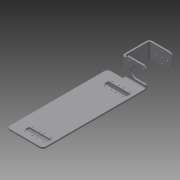
# Autodesk Inventor part: Base
Saved by Autodesk Inventor 2015 (Build 190159000, 159)
## iProperties
Created: 2015-12-09
Part Number: Base
Material: Generic
Document SubType Name: Sheet Metal
Designer: Nick
Density: 1 g/cm^3
Sheet Metal Rule: Default
Appearance: Default
Author: Nick
Autodesk Inventor part; units mm, degrees
ref_plane "YZ Plane" through (0, 0, 0) normal (1, 0, 0) x (0, 1, 0)
ref_plane "XZ Plane" through (0, 0, 0) normal (0, 1, 0) x (-1, 0, 0)
ref_plane "XY Plane" through (0, 0, 0) normal (0, 0, 1) x (1, 0, 0)
sketch "Sketch1" plane through (0, 0, 0) normal (0, 1, 0) x (-1, 0, 0)
  line L0 (0, 0) -> (0, -208.3054)
  line L1 (0, 0) -> (0, 0)
  line L2 (6.35, 6.35) -> (6.35, 6.35)
  line L3 (6.35, 6.35) -> (70.4596, 6.35)
  line L4 (70.4596, 6.35) -> (76.8096, 6.35)
  line L5 (76.8096, 0) -> (76.8096, -201.9554)
  line L6 (76.8096, -208.3054) -> (70.4596, -208.3054)
  line L7 (70.4596, -208.3054) -> (43.6118, -208.3054)
  line L8 (43.6118, -208.3054) -> (43.6118, -217.6526)
  line L9 (43.6118, -217.6526) -> (43.6118, -249.9614)
  line L10 (0, -208.3054) -> (0, -217.6526)
  line L11 (0, -217.6526) -> (43.6118, -217.6526)
  line L12 (0, -208.3054) -> (43.6118, -208.3054)
  line L13 (43.6118, -212.979) -> (0, -212.979)
  arc A0 (70.4596, -208.3054) -> (76.8096, -201.9554) centre (70.4596, -201.9554) ccw
  arc A1 (76.8096, 0) -> (70.4596, 6.35) centre (70.4596, 0) ccw
  arc A2 (6.35, 6.35) -> (0, 0) centre (6.35, 0) ccw
  line L14 (43.6118, -249.9614) -> (43.6118, -253.9492)
  line L15 (0, -253.9492) -> (0, -249.9614)
  line L16 (0, -249.9614) -> (43.6118, -249.9614)
  line L17 (0, -249.9614) -> (0, -217.6526)
  circle A3 centre (20.574, -232.791) radius 12.7
  line L18 (20.574, -245.491) -> (0, -245.491)
  line L19 (20.574, -220.091) -> (0, -220.091)
  line L20 (0, -249.9614) -> (3.9878, -253.9492)
  line L21 (43.6118, -249.9614) -> (39.624, -253.9492)
  line L22 (3.9878, -253.9492) -> (39.624, -253.9492)
  circle A4 centre (5.9436, -248.3104) radius 1.4859
  line L23 (5.9436, -248.3104) -> (36.3728, -248.3104)
  circle A5 centre (36.3728, -248.3104) radius 1.4859
  line L24 (43.6118, -217.6526) -> (52.959, -217.6526)
  line L25 (52.959, -217.6526) -> (52.959, -249.9614)
  line L26 (52.959, -249.9614) -> (43.6118, -249.9614)
  line L27 (48.2854, -249.9614) -> (48.2854, -217.6526)
  line L28 (52.959, -217.6526) -> (96.9518, -217.6526)
  line L29 (96.9518, -217.6526) -> (96.9518, -249.9614)
  line L30 (96.9518, -249.9614) -> (52.959, -249.9614)
  line L31 (96.9518, -249.9614) -> (106.299, -249.9614)
  line L32 (106.299, -249.9614) -> (106.299, -217.6526)
  line L33 (106.299, -217.6526) -> (96.9518, -217.6526)
  line L34 (101.6254, -217.6526) -> (101.6254, -249.9614)
  line L35 (106.299, -217.6526) -> (143.5608, -217.6526)
  line L36 (143.5608, -217.6526) -> (143.5608, -249.9614)
  line L37 (143.5608, -249.9614) -> (106.299, -249.9614)
  line L38 (143.5608, -249.9614) -> (143.5608, -249.9614)
  line L39 (149.9108, -243.6114) -> (149.9108, -224.0026)
  line L40 (143.5608, -217.6526) -> (143.5608, -217.6526)
  arc A6 (149.9108, -224.0026) -> (143.5608, -217.6526) centre (143.5608, -224.0026) ccw
  arc A7 (143.5608, -249.9614) -> (149.9108, -243.6114) centre (143.5608, -243.6114) ccw
  circle A8 centre (128.8542, -233.807) radius 1.9939
  circle A9 centre (117.5512, -233.807) radius 1.4859
  circle A10 centre (128.8542, -245.11) radius 1.4859
  circle A11 centre (140.1572, -233.807) radius 1.4859
  circle A12 centre (128.8542, -222.504) radius 1.4859
  line L41 (0, -208.3054) -> (70.4596, -208.3054)
  arc A13 (70.4596, -208.3054) -> (76.8096, -201.9554) centre (70.4596, -201.9554) ccw
  line L42 (43.6118, -249.9614) -> (39.624, -253.9492)
  line L43 (3.9878, -253.9492) -> (39.624, -253.9492)
  line L44 (0, -249.9614) -> (3.9878, -253.9492)
  line L45 (0, -249.9614) -> (43.6118, -249.9614)
  line L46 (5.9944, -9.398) -> (5.9944, -18.4912)
  line L47 (5.9944, -18.4912) -> (53.8988, -18.4912)
  line L48 (53.8988, -18.4912) -> (53.8988, -9.398)
  line L49 (53.8988, -9.398) -> (5.9944, -9.398)
  line L50 (9.2964, -6.7056) -> (11.8872, -6.7056)
  line L51 (11.8872, -6.7056) -> (11.8872, -5.1562)
  line L52 (11.8872, -5.1562) -> (9.2964, -5.1562)
  line L53 (9.2964, -5.1562) -> (9.2964, -6.7056)
  line L54 (23.9268, -6.7056) -> (26.5176, -6.7056)
  line L55 (26.5176, -6.7056) -> (26.5176, -5.1562)
  line L56 (26.5176, -5.1562) -> (23.9268, -5.1562)
  line L57 (23.9268, -5.1562) -> (23.9268, -6.7056)
  line L58 (29.9466, -9.398) -> (29.9466, -18.4912)
  line L59 (53.8988, -13.9446) -> (41.6179, -13.9446)
  line L60 (50.5968, -6.7056) -> (48.006, -6.7056)
  line L61 (48.006, -6.7056) -> (48.006, -5.1562)
  line L62 (48.006, -5.1562) -> (50.5968, -5.1562)
  line L63 (50.5968, -5.1562) -> (50.5968, -6.7056)
  line L64 (35.9664, -6.7056) -> (33.3756, -6.7056)
  line L65 (33.3756, -6.7056) -> (33.3756, -5.1562)
  line L66 (33.3756, -5.1562) -> (35.9664, -5.1562)
  line L67 (35.9664, -5.1562) -> (35.9664, -6.7056)
  line L68 (9.2964, -21.1836) -> (11.8872, -21.1836)
  line L69 (11.8872, -21.1836) -> (11.8872, -22.733)
  line L70 (11.8872, -22.733) -> (9.2964, -22.733)
  line L71 (9.2964, -22.733) -> (9.2964, -21.1836)
  line L72 (23.9268, -21.1836) -> (26.5176, -21.1836)
  line L73 (26.5176, -21.1836) -> (26.5176, -22.733)
  line L74 (26.5176, -22.733) -> (23.9268, -22.733)
  line L75 (23.9268, -22.733) -> (23.9268, -21.1836)
  line L76 (50.5968, -22.733) -> (50.5968, -21.1836)
  line L77 (48.006, -22.733) -> (50.5968, -22.733)
  line L78 (50.5968, -21.1836) -> (48.006, -21.1836)
  line L79 (48.006, -21.1836) -> (48.006, -22.733)
  line L80 (35.9664, -22.733) -> (35.9664, -21.1836)
  line L81 (33.3756, -22.733) -> (35.9664, -22.733)
  line L82 (35.9664, -21.1836) -> (33.3756, -21.1836)
  line L83 (33.3756, -21.1836) -> (33.3756, -22.733)
  line L84 (5.9944, -18.4912) -> (5.9944, -178.2064)
  line L85 (5.9944, -98.3488) -> (43.6118, -98.3488)
  line L86 (5.9944, -187.2996) -> (5.9944, -178.2064)
  line L87 (5.9944, -178.2064) -> (53.8988, -178.2064)
  line L88 (53.8988, -178.2064) -> (53.8988, -187.2996)
  line L89 (53.8988, -187.2996) -> (5.9944, -187.2996)
  line L90 (9.2964, -189.992) -> (11.8872, -189.992)
  line L91 (11.8872, -189.992) -> (11.8872, -191.5414)
  line L92 (11.8872, -191.5414) -> (9.2964, -191.5414)
  line L93 (9.2964, -191.5414) -> (9.2964, -189.992)
  line L94 (23.9268, -189.992) -> (26.5176, -189.992)
  line L95 (26.5176, -189.992) -> (26.5176, -191.5414)
  line L96 (26.5176, -191.5414) -> (23.9268, -191.5414)
  line L97 (23.9268, -191.5414) -> (23.9268, -189.992)
  line L98 (29.9466, -187.2996) -> (29.9466, -178.2064)
  line L99 (53.8988, -182.753) -> (41.6179, -182.753)
  line L100 (50.5968, -191.5414) -> (50.5968, -189.992)
  line L101 (48.006, -191.5414) -> (50.5968, -191.5414)
  line L102 (50.5968, -189.992) -> (48.006, -189.992)
  line L103 (48.006, -189.992) -> (48.006, -191.5414)
  line L104 (35.9664, -191.5414) -> (35.9664, -189.992)
  line L105 (33.3756, -191.5414) -> (35.9664, -191.5414)
  line L106 (35.9664, -189.992) -> (33.3756, -189.992)
  line L107 (33.3756, -189.992) -> (33.3756, -191.5414)
  line L108 (23.9268, -175.514) -> (26.5176, -175.514)
  line L109 (26.5176, -173.9646) -> (23.9268, -173.9646)
  line L110 (23.9268, -173.9646) -> (23.9268, -175.514)
  line L111 (11.8872, -175.514) -> (11.8872, -173.9646)
  line L112 (9.2964, -175.514) -> (11.8872, -175.514)
  line L113 (11.8872, -173.9646) -> (9.2964, -173.9646)
  line L114 (9.2964, -173.9646) -> (9.2964, -175.514)
  line L115 (26.5176, -175.514) -> (26.5176, -173.9646)
  line L116 (35.9664, -175.514) -> (33.3756, -175.514)
  line L117 (33.3756, -175.514) -> (33.3756, -173.9646)
  line L118 (33.3756, -173.9646) -> (35.9664, -173.9646)
  line L119 (35.9664, -173.9646) -> (35.9664, -175.514)
  line L120 (48.006, -175.514) -> (48.006, -173.9646)
  line L121 (50.5968, -173.9646) -> (50.5968, -175.514)
  line L122 (48.006, -173.9646) -> (50.5968, -173.9646)
  line L123 (50.5968, -175.514) -> (48.006, -175.514)
  line L124 (5.9944, -178.2064) -> (5.9944, -18.4912)
  point P0 (0, 6.35)
  point P1 (149.9108, -249.9614)
  point P2 (149.9108, -217.6526)
  point P3 (149.9108, -233.807)
  dimension "d0" = 208.3054
  dimension "d1" = 6.35
  dimension "d2" = 6.35
  dimension "d3" = 64.1096
  dimension "d4" = 6.35
  dimension "d5" = 6.35
  dimension "d6" = 26.8478
  dimension "d7" = 9.3472
  dimension "d8" = 32.3088
  dimension "d9" = 9.3472
  dimension "d10" = 6.35
  dimension "d11" = 3.9878
  dimension "d12" = 3.9878
  dimension "d13" = 25.4
  dimension "d14" = 20.574
  dimension "d16" = 15.1384
  dimension "d17" = 3.9878
  dimension "d18" = 0
  dimension "d19" = 3.9878
  dimension "d20" = 2.9718
  dimension "d21" = 5.9436
  dimension "d22" = 5.6388
  dimension "d23" = 30.4292
  dimension "d24" = 2.9718
  dimension "d25" = 2.4384
  dimension "d26" = 25.4
  dimension "d27" = 32.3088
  dimension "d28" = 3.9878
  dimension "d29" = 9.3472
  dimension "d30" = 43.9928
  dimension "d31" = 9.3472
  dimension "d32" = 37.2618
  dimension "d33" = 6.35
  dimension "d34" = 6.35
  dimension "d35" = 21.0566
  dimension "d36" = 0
  dimension "d37" = 3.9878
  dimension "d38" = 2.9718
  dimension "d39" = 11.303
  dimension "d42" = 360
  dimension "d44" = 15.748
  dimension "d45" = 5.9944
  dimension "d46" = 9.0932
  dimension "d47" = 47.9044
  dimension "d48" = 2.6924
  dimension "d49" = 3.302
  dimension "d50" = 2.5908
  dimension "d51" = 1.5494
  dimension "d52" = 12.0396
  dimension "d53" = 2.5908
  dimension "d54" = 0
  dimension "d55" = 0
  dimension "d56" = 159.7152
  constraints: 250 end point, 65 symmetric about line, 24 point on line, 22 perpendicular, 14 centre point, 14 point on circle, 11 midpoint, 10 tangent, 8 horizontal, 6 coincident, 6 vertical, 4 equal radius, 4 parallel, 2 collinear, 11 other
  measures "d0" distance of L0.start L0.end
  measures "d1" distance of L0.start point (0, 6.35)
  measures "d2" distance of point (0, 6.35) L2.end
  measures "d3" distance of L2.end L4.start
  measures "d4" distance of L4.start L4.end
  measures "d5" distance of L6.start L6.end
  measures "d6" distance of L6.end L7.end
  measures "d7" distance of L7.end L8.end
  measures "d8" distance of L8.end L9.end
  measures "d9" distance of L0.end L10.end
  measures "d10" radius of A0
  measures "d11" distance of L9.end L14.end
  measures "d12" distance of L15.start L15.end
  measures "d13" diameter of A3
  measures "d14" distance from line of L17 A3.centre
  measures "d16" distance from line of L11 A3.centre
  measures "d17" distance from line of L14 L21.end
  measures "d18" distance of L20.end L22.start
  measures "d19" distance of L15.start L22.start
  measures "d20" diameter of A4
  measures "d21" distance from line of L17 L23.start
  measures "d22" distance from line of L22 L23.start
  measures "d23" distance of L23.start L23.end
  measures "d24" diameter of A5
  measures "d25" distance between parallel lines of L11 L19
  measures "d26" distance between parallel lines of L19 L18
  measures "d27" distance of L15.end L10.end
  measures "d28" distance from line of L15.end L22
  measures "d29" distance of L8.end L24.end
  measures "d30" distance of L24.end L28.end
  measures "d31" distance of L29.end L31.end
  measures "d32" distance of L32.end L35.end
  measures "d33" distance of L36.end point (149.911, -249.961)
  measures "d34" radius of A6
  measures "d35" distance from line of L39 point (128.854, -233.807)
  measures "d36" vertical distance of point (128.854, -233.807) point (149.911, -233.807)
  measures "d37" diameter of A8
  measures "d38" diameter of A9
  measures "d39" distance of point (128.854, -233.807) point (117.551, -233.807)
  measures "d44" distance from line of L3 L46.start
  measures "d45" distance from line of L0 L46.start
  measures "d46" distance of L46.start L46.end
  measures "d47" distance of L46.end L47.end
  measures "d48" vertical distance of L46.start L50.start
  measures "d49" horizontal distance of L46.start L50.start
  measures "d50" distance of L52.end L51.end
  measures "d51" distance of L51.end L50.end
  measures "d52" distance from line of L51 L54.start
  measures "d53" distance of L56.end L55.end
  measures "d54" distance from line of L50 L54.start
  measures "d55" distance between parallel lines of L52 L56
  measures "d56" distance of L46.end L84.end
extrude "Plate1" add sketch "Sketch1" along normal blind 3.048 contours A2 L3 A1 L5 A0 L7 L12 L0 | L12 L8 L13 L10 | L13 L8 L11 L10 | L11 L9 L16 L17 L18 A3 L19 | L24 L27 L26 L9 | L21 L22 L20 L16 | L24 L25 L26 L27 | L28 L29 L30 L25 | L33 L34 L31 L29 | L33 L32 L31 L34 | L35 L36 L37 L32 | A6 L39 A7 L36
fold "Fold1" angle 90 bend radius 3.048 thickness 3.048 k factor 0.44 line from (-101.6254, 0, -217.6526) to (-101.6254, 0, -249.9614) line at bend centre moving side (-1, 0, 0) folds toward (0, -1, 0)
fold "Fold2" angle 90 bend radius 3.048 thickness 3.048 k factor 0.44 line from (-48.2854, 0, -249.9614) to (-48.2854, 0, -217.6526) line at bend centre moving side (-1, 0, 0) folds toward (0, -1, 0)
fold "Fold3" angle 90 bend radius 3.048 thickness 3.048 k factor 0.44 line from (-43.6118, 0, -212.979) to (0, 0, -212.979) line at bend centre moving side (0, 0, -1) folds toward (0, 1, 0)
equation "\"d58\" = BendReliefWidth"
equation "\"d59\" = BendReliefDepth"
equation "\"d60\" = MinimumRemnant"
equation "\"d61\" = BendRadius"
equation "\"d63\" = BendRadius"
equation "\"d64\" = BendReliefWidth"
equation "\"d65\" = BendReliefDepth"
equation "\"d66\" = MinimumRemnant"
equation "\"d67\" = BendRadius"
equation "\"d69\" = BendRadius"
equation "\"d70\" = BendReliefWidth"
equation "\"d71\" = BendReliefDepth"
equation "\"d72\" = MinimumRemnant"
equation "\"d73\" = BendRadius"
equation "\"d75\" = BendRadius"
equation "\"BendRadius\" = Thickness"
equation "\"BendReliefWidth\" = Thickness"
equation "\"BendReliefDepth\" = 0.5 * Thickness"
equation "\"CornerReliefSize\" = 4 * Thickness"
equation "\"MinimumRemnant\" = 2 * Thickness"
equation "\"TransitionRadius\" = BendRadius"
equation "\"JacobiRadiusSize\" = BendRadius"
equation "\"GapSize\" = Thickness"
equation "\"d57\" = BendRadius"
equation "\"Thickness\" = 3.048"
body "Solid1"
